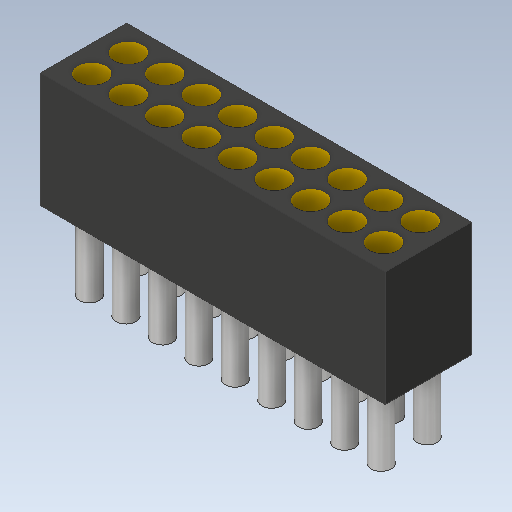
# Autodesk Inventor part: Millmax
Saved by Autodesk Inventor 2020 (Build 240168000, 168)
## iProperties
Created: 2019-02-19
Part Number: Millmax
Material: 일반
Document SubType Name: Modeling
Designer: Jeong Ji Hoon
Density: 1 g/cm^3
Appearance: 기본값
Author: Jeong Ji Hoon
Autodesk Inventor part; units mm, degrees
ref_plane "YZ Plane" through (0, 0, 0) normal (1, 0, 0) x (0, 1, 0)
ref_plane "XZ Plane" through (0, 0, 0) normal (0, 1, 0) x (-1, 0, 0)
ref_plane "XY Plane" through (0, 0, 0) normal (0, 0, 1) x (1, 0, 0)
sketch "스케치1" plane through (0, 0, 0) normal (0, 1, 0) x (-1, 0, 0)
  line L0 (0, 0) -> (12, 0)
  line L1 (12, 0) -> (12, -3)
  line L2 (12, -3) -> (0, -3)
  line L3 (0, -3) -> (0, 0)
  dimension "d0" = 12
  dimension "d1" = 3
  constraints: 8 end point, 2 parallel, 1 horizontal, 1 perpendicular
  measures "d0" distance of L1.end L2.end
  measures "d1" distance of L0.end L1.end
extrude "돌출1" add sketch "스케치1" along normal blind 4
sketch "스케치2" plane through (0, 4, 0) normal (0, 1, 0) x (1, 0, 0)
  line L0 (-12, 0) -> (0, 0) projected
  line L1 (0, 0) -> (0, 3) projected
  line L2 (0, 3) -> (-12, 3) projected
  line L3 (-12, 3) -> (-12, 0) projected
  point P0 (-11.08, 0.865)
  point P1 (-9.81, 0.865)
  point P2 (-8.54, 0.865)
  point P3 (-7.27, 0.865)
  point P4 (-6, 0.865)
  point P5 (-4.73, 0.865)
  point P6 (-3.46, 0.865)
  point P7 (-2.19, 0.865)
  point P8 (-0.92, 0.865)
  point P9 (-11.08, 2.135)
  point P10 (-9.81, 2.135)
  point P11 (-8.54, 2.135)
  point P12 (-7.27, 2.135)
  point P13 (-6, 2.135)
  point P14 (-4.73, 2.135)
  point P15 (-3.46, 2.135)
  point P16 (-2.19, 2.135)
  point P17 (-0.92, 2.135)
  dimension "d6" = 1.27
  dimension "d9" = 1.27
  dimension "d12" = 0.865
  dimension "d13" = 0.865
  dimension "d14" = 0.92
  dimension "d15" = 0.92
  constraints: 1 horizontal, 1 vertical, 17 other
  measures "d6" distance of point (-11.08, 0.865) point (-9.81, 0.865)
  measures "d9" distance of point (-11.08, 0.865) point (-11.08, 2.135)
  measures "d12" distance from line of L0 point (-11.08, 0.865)
  measures "d13" distance from line of L2 point (-11.08, 2.135)
  measures "d14" distance from line of L3 point (-11.08, 2.135)
  measures "d15" distance from line of point (-0.92, 2.135) L1
hole "구멍1" at (-11.08, 4, -0.865) at (-9.81, 4, -0.865) at (-8.54, 4, -0.865) at (-7.27, 4, -0.865) at (-6, 4, -0.865) at (-4.73, 4, -0.865) at (-3.46, 4, -0.865) at (-2.19, 4, -0.865) at (-0.92, 4, -0.865) at (-11.08, 4, -2.135) at (-9.81, 4, -2.135) at (-8.54, 4, -2.135) at (-7.27, 4, -2.135) at (-6, 4, -2.135) at (-4.73, 4, -2.135) at (-3.46, 4, -2.135) at (-2.19, 4, -2.135) at (-0.92, 4, -2.135) direction (0, -1, 0) diameter 1 depth 2
sketch "스케치3" plane through (0, 0, 0) normal (0, -1, 0) x (1, 0, 0)
  circle A0 centre (-2.19, -2.135) radius 0.5 projected
  circle A1 centre (-4.73, -2.135) radius 0.5 projected
  circle A2 centre (-7.27, -2.135) radius 0.5 projected
  circle A3 centre (-9.81, -2.135) radius 0.5 projected
  circle A4 centre (-0.92, -0.865) radius 0.5 projected
  circle A5 centre (-3.46, -0.865) radius 0.5 projected
  circle A6 centre (-6, -0.865) radius 0.5 projected
  circle A7 centre (-8.54, -0.865) radius 0.5 projected
  circle A8 centre (-11.08, -0.865) radius 0.5 projected
  circle A9 centre (-9.81, -0.865) radius 0.5 projected
  circle A10 centre (-7.27, -0.865) radius 0.5 projected
  circle A11 centre (-4.73, -0.865) radius 0.5 projected
  circle A12 centre (-2.19, -0.865) radius 0.5 projected
  circle A13 centre (-11.08, -2.135) radius 0.5 projected
  circle A14 centre (-8.54, -2.135) radius 0.5 projected
  circle A15 centre (-6, -2.135) radius 0.5 projected
  circle A16 centre (-3.46, -2.135) radius 0.5 projected
  circle A17 centre (-0.92, -2.135) radius 0.5 projected
  line L0 (-12, 0) -> (0, 0) projected
  line L1 (0, 0) -> (0, -3) projected
  line L2 (0, -3) -> (-12, -3) projected
  line L3 (-12, -3) -> (-12, 0) projected
  circle A18 centre (-11, -2.3) radius 0.35
  circle A19 centre (-9.73, -2.3) radius 0.35
  circle A20 centre (-8.46, -2.3) radius 0.35
  circle A21 centre (-7.19, -2.3) radius 0.35
  circle A22 centre (-5.92, -2.3) radius 0.35
  circle A23 centre (-4.65, -2.3) radius 0.35
  circle A24 centre (-3.38, -2.3) radius 0.35
  circle A25 centre (-2.11, -2.3) radius 0.35
  circle A26 centre (-0.84, -2.3) radius 0.35
  circle A27 centre (-11, -0.7) radius 0.35
  circle A28 centre (-9.73, -0.7) radius 0.35
  circle A29 centre (-8.46, -0.7) radius 0.35
  circle A30 centre (-7.19, -0.7) radius 0.35
  circle A31 centre (-5.92, -0.7) radius 0.35
  circle A32 centre (-4.65, -0.7) radius 0.35
  circle A33 centre (-3.38, -0.7) radius 0.35
  circle A34 centre (-2.11, -0.7) radius 0.35
  circle A35 centre (-0.84, -0.7) radius 0.35
  dimension "d23" = 1.27
  dimension "d24" = 0.7
  dimension "d27" = 1.27
  dimension "d30" = 1.6
  dimension "d33" = 0.9
  dimension "d34" = 0.7
  dimension "d35" = 0.7
  dimension "d36" = 1
  constraints: 18 centre point, 1 horizontal, 1 vertical, 34 other
  measures "d23" distance of A8.centre A13.centre
  measures "d24" diameter of A18
  measures "d27" distance of A18.centre A19.centre
  measures "d30" distance of A18.centre A27.centre
  measures "d34" distance from line of L2 A18.centre
  measures "d35" distance from line of L0 A27.centre
  measures "d36" distance from line of L3 A18.centre
extrude "돌출2" add sketch "스케치3" along normal blind 2.54 separate body contours A25 A0 | A0 A25 | A23 A1 | A1 A23 | A21 A2 | A2 A21 | A19 A3 | A3 A19 | A35 A4 | A4 A35 | A33 A5 | A5 A33 | A31 A6 | A6 A31 | A29 A7 | A7 A29 | A27 A8 | A8 A27 | A28 A9 | A9 A28 | A30 A10 | A10 A30 | A32 A11 | A11 A32 | A34 A12 | A12 A34 | A18 A13 | A13 A18 | A20 A14 | A14 A20 | A22 A15 | A15 A22 | A24 A16 | A16 A24 | A26 A17 | A17 A26 picked at (-2.1777, -2.1932) picked at (-1.9214, -2.5663) picked at (-4.7177, -2.1932) picked at (-4.4614, -2.5663) picked at (-7.2577, -2.1932) picked at (-7.0014, -2.5663) picked at (-9.7977, -2.1932) picked at (-9.5414, -2.5663) picked at (-0.9077, -0.8068) picked at (-0.6514, -0.4337) picked at (-3.4477, -0.8068) picked at (-3.1914, -0.4337) picked at (-5.9877, -0.8068) picked at (-5.7314, -0.4337) picked at (-8.5277, -0.8068) picked at (-8.2714, -0.4337) picked at (-11.0677, -0.8068) picked at (-10.9077, -0.387) picked at (-9.7977, -0.8068) picked at (-9.6377, -0.387) picked at (-7.2577, -0.8068) picked at (-7.0014, -0.4337) picked at (-4.7177, -0.8068) picked at (-4.4614, -0.4337) picked at (-2.1777, -0.8068) picked at (-2.0177, -0.387) picked at (-11.0677, -2.1932) picked at (-10.8114, -2.5663) picked at (-8.5277, -2.1932) picked at (-8.2714, -2.5663) picked at (-5.9877, -2.1932) picked at (-5.7314, -2.5663) picked at (-3.4477, -2.1932) picked at (-3.1914, -2.5663) picked at (-0.9077, -2.1932) picked at (-0.6514, -2.5663)
equation "\"d14\" = d15"
